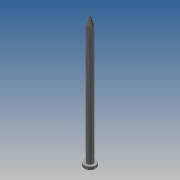
# Autodesk Inventor part: nail
Saved by Autodesk Inventor 2013 SP2 (Build 170200200, 200)
## iProperties
Created: 2013-05-14
Part Number: nail
Material: Steel, Galvanized
Document SubType Name: Modeling
Designer: Dave
Density: 7.85 g/cm^3
Mass: 4.67275 g
Surface Area: 9.24741 cm^2
Volume: 0.595255 cm^3
Author: Dave
Autodesk Inventor part; units mm, degrees
ref_plane "YZ Plane" through (0, 0, 0) normal (1, 0, 0) x (0, 1, 0)
ref_plane "XZ Plane" through (0, 0, 0) normal (0, 1, 0) x (-1, 0, 0)
sketch "Sketch1" plane through (0, 0, 0) normal (0, 1, 0) x (-1, 0, 0)
  circle A0 centre (0, 0) radius 4.445
  dimension "d0" = 8.89
  constraints: 1 centre point, 1 coincident
  measures "d0" diameter of A0
extrude "Extrusion1" add sketch "Sketch1" along normal blind 2.54
sketch "Sketch2" plane through (0, 2.54, 0) normal (0, 1, 0) x (1, 0, 0)
  circle A0 centre (0, 0) radius 4.445 projected
  circle A1 centre (0, 0) radius 2.4384
  dimension "d5" = 4.8768
  constraints: 1 centre point, 1 coincident
  measures "d5" diameter of A1
extrude "Extrusion2" add sketch "Sketch2" along normal blind 101.6 contours A1
sketch "Sketch3" plane through (0, 104.14, 0) normal (0, 1, 0) x (1, 0, 0)
  circle A0 centre (0, 0) radius 2.4384 projected
  point P0 (0, 2.4384)
  constraints: 1 vertical alignment, 1 other
ref_plane "Work Plane2" through (0, 104.14, 0) normal (0, 0, -1) x (-1, 0, 0)
ref_plane "Work Plane1" through (0, 104.14, -2.4384) normal (0, 0, -1) x (-1, 0, 0)
sketch "Sketch4" plane through (0, 104.14, 0) normal (0, 0, -1) x (-1, 0, 0)
  line L0 (3.175, -4.7625) -> (3.175, 0)
  line L1 (3.175, 0) -> (0, 0)
  line L2 (0, 0.1023) -> (0, 1.7624)
  line L3 (0, 0) -> (3.175, -9.525)
  line L4 (3.175, -4.7625) -> (3.175, -9.525)
  point P0 (0, -104.14)
  constraints: 10 end point, 2 perpendicular, 1 parallel, 1 vertical
revolve "Revolution1" cut sketch "Sketch4" angle 360 about axis through (0, 104.2423, 0) along (0, 1, 0)
fillet "Fillet1" radius 0.508 1 edges at (4.445, 0, 0)
body "Solid1"
